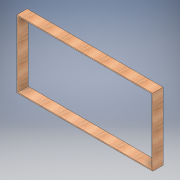
# Autodesk Inventor part: Frame
Saved by Autodesk Inventor 2019.3 (Build 233278000, 278)
## iProperties
Created: 2020-08-13
Part Number: Frame
Material: Holz (Birke)
Document SubType Name: Modeling
Designer: Nicolas Frick
Density: 0.55 g/cm^3
Appearance: Birke - natur - poliert
Author: Nicolas Frick
Autodesk Inventor part; units mm, degrees
ref_plane "YZ Plane" through (0, 0, 0) normal (1, 0, 0) x (0, 1, 0)
ref_plane "XZ Plane" through (0, 0, 0) normal (0, 1, 0) x (-1, 0, 0)
ref_plane "XY Plane" through (0, 0, 0) normal (0, 0, 1) x (1, 0, 0)
sketch "Skizze1" plane through (0, 0, 0) normal (0, 0, 1) x (1, 0, 0)
  line L0 (-914, 455) -> (914, 455)
  line L1 (914, 455) -> (914, -455)
  line L2 (914, -455) -> (-914, -455)
  line L3 (-914, -455) -> (-914, 455)
  line L4 (-914, 455) -> (914, -455) construction
  line L5 (914, 455) -> (-914, -455) construction
  line L6 (-901.5, -442.5) -> (901.5, -442.5)
  line L7 (901.5, -442.5) -> (901.5, 442.5)
  line L8 (901.5, 442.5) -> (-901.5, 442.5)
  line L9 (-901.5, 442.5) -> (-901.5, -442.5)
  line L10 (-901.5, -442.5) -> (901.5, 442.5) construction
  line L11 (901.5, -442.5) -> (-901.5, 442.5) construction
  point P0 (0, 0)
  dimension "d0" = 1828
  dimension "d1" = 910
  dimension "d2" = 1803
  dimension "d3" = 885
  constraints: 24 end point, 4 midpoint, 4 parallel, 2 horizontal, 2 perpendicular
  measures "d0" distance of L1.end L2.end
  measures "d1" distance of L0.end L1.end
  measures "d2" distance of L8.end L7.end
  measures "d3" distance of L7.end L6.end
extrude "Extrusion1" add sketch "Skizze1" along normal blind 139
sketch "Skizze2" plane through (0, 0, 139) normal (0, 0, 1) x (1, 0, 0)
  line L0 (-901.5, 442.5) -> (901.5, 442.5) projected
  line L1 (-901.5, -442.5) -> (-901.5, 442.5) projected
  line L2 (901.5, -442.5) -> (-901.5, -442.5) projected
  line L3 (901.5, 442.5) -> (901.5, -442.5) projected
  point P0 (0, 0)
